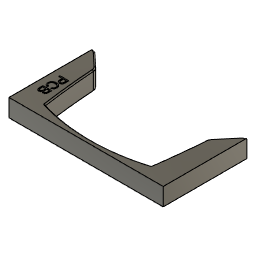
pcb_Dispensor_holder (Autodesk Fusion 360 design; units mm, degrees)
Autodesk Fusion 360 part; units mm, degrees
sketch "Sketch1" plane through (0, 0, 0) normal (0, 0, 1) x (1, 0, 0)
  line L0 (0, 0) -> (70, 0)
  line L1 (70, 0) -> (70, 70)
  line L2 (70, 70) -> (0, 70)
  line L3 (0, 70) -> (0, 0)
  line L4 (35, 0) -> (35, 2)
  spline S0 degree 5 poles (10.999997, 5.500001) (11.155561, 5.453683) (11.466888, 5.361799) (11.934471, 5.226228) (12.559102, 5.049976) (13.341865, 4.83719) (14.126594, 4.631952) (14.913263, 4.43428) (15.70183, 4.244194) (16.492223, 4.061708) (17.284358, 3.886836) (18.078142, 3.719588) (18.873486, 3.559975) (19.670315, 3.408007) (20.468575, 3.263698) (21.268224, 3.127064) (22.069221, 2.998132) (22.871516, 2.876939) (23.675037, 2.76354) (24.479682, 2.658009) (25.285329, 2.560422) (26.091853, 2.470835) (26.899136, 2.389272) (27.707084, 2.3157) (28.515633, 2.250011) (29.324747, 2.192062) (30.134393, 2.141705) (30.944536, 2.098828) (31.755125, 2.063387) (32.566073, 2.035442) (33.377278, 2.015122) (34.188626, 2.002585) (35.000008, 1.997988) (35.811324, 2.001442) (36.622501, 2.012982) (37.433482, 2.032584) (38.244219, 2.060187) (39.054663, 2.095711) (39.864763, 2.139079) (40.674451, 2.190236) (41.483649, 2.249147) (42.292272, 2.315789) (43.100227, 2.390151) (43.907418, 2.472228) (44.713752, 2.562017) (45.519136, 2.659519) (46.323491, 2.764743) (47.126755, 2.877707) (47.928887, 2.998437) (48.729875, 3.126975) (49.529715, 3.263365) (50.328395, 3.407636) (51.125872, 3.559798) (51.922055, 3.719827) (52.716787, 3.887649) (53.509869, 4.063161) (54.301082, 4.246242) (55.090222, 4.436771) (55.877114, 4.634637) (56.661648, 4.839761) (57.443758, 5.052087) (58.067484, 5.227679) (58.534171, 5.36259) (58.844804, 5.453959) (58.999997, 5.500001) knots 0 0 0 0 0 0 0.01666667 0.03333333 0.05 0.06666667 0.08333333 0.1 0.11666667 0.13333333 0.15 0.16666667 0.18333333 0.2 0.21666667 0.23333333 0.25 0.26666667 0.28333333 0.3 0.31666667 0.33333333 0.35 0.36666667 0.38333333 0.4 0.41666667 0.43333333 0.45 0.46666667 0.48333333 0.5 0.51666667 0.53333333 0.55 0.56666667 0.58333333 0.6 0.61666667 0.63333333 0.65 0.66666667 0.68333333 0.7 0.71666667 0.73333333 0.75 0.76666667 0.78333333 0.8 0.81666667 0.83333333 0.85 0.86666667 0.88333333 0.9 0.91666667 0.93333333 0.95 0.96666667 0.98333333 1 1 1 1 1 1
  spline S1 degree 5 poles (58.999997, 5.500001) (59.01455, 5.602527) (59.04395, 5.810642) (59.088931, 6.131994) (59.150678, 6.578903) (59.230393, 7.164734) (59.311475, 7.767981) (59.391329, 8.366775) (59.466575, 8.932747) (59.535207, 9.449558) (59.598272, 9.92737) (59.66196, 10.420796) (59.73467, 11.003713) (59.824179, 11.745021) (59.934208, 12.679149) (60.063255, 13.795991) (60.206503, 15.057047) (60.356952, 16.404923) (60.506823, 17.775214) (60.64889, 19.107692) (60.777733, 20.356871) (60.891317, 21.505277) (60.990565, 22.559989) (61.078304, 23.543942) (61.158448, 24.48917) (61.235067, 25.429138) (61.311554, 26.391886) (61.389627, 27.391781) (61.469549, 28.431304) (61.550566, 29.504582) (61.631253, 30.600245) (61.709907, 31.704562) (61.784901, 32.804352) (61.855087, 33.890205) (61.919728, 34.956001) (61.978402, 35.998148) (62.020415, 36.811581) (62.049133, 37.41002) (62.067038, 37.803816) (62.075682, 37.999422) knots 0 0 0 0 0 0 0.02857143 0.05714286 0.08571429 0.11428571 0.14285714 0.17142857 0.2 0.22857143 0.25714286 0.28571429 0.31428571 0.34285714 0.37142857 0.4 0.42857143 0.45714286 0.48571429 0.51428571 0.54285714 0.57142857 0.6 0.62857143 0.65714286 0.68571429 0.71428571 0.74285714 0.77142857 0.8 0.82857143 0.85714286 0.88571429 0.91428571 0.94285714 0.97142857 1 1 1 1 1 1
  spline S2 degree 5 poles (10.999997, 5.500001) (10.95489, 5.823121) (10.865295, 6.469506) (10.732765, 7.439517) (10.559793, 8.733734) (10.349927, 10.352962) (10.146623, 11.973629) (9.950184, 13.595674) (9.761002, 15.218964) (9.579547, 16.843273) (9.406299, 18.468328) (9.241664, 20.093857) (9.085891, 21.719638) (8.938976, 23.345548) (8.800554, 24.971608) (8.670024, 26.597942) (8.546659, 28.224733) (8.429709, 29.85218) (8.318502, 31.480453) (8.212533, 33.109654) (8.111452, 34.739832) (8.034323, 36.044766) (7.978526, 37.023912) (7.942236, 37.676872) (7.924318, 38.003401) knots 0 0 0 0 0 0 0.05 0.1 0.15 0.2 0.25 0.3 0.35 0.4 0.45 0.5 0.55 0.6 0.65 0.7 0.75 0.8 0.85 0.9 0.95 1 1 1 1 1 1
  line L5 (7.924318, 38.003401) -> (0, 38.003401)
  line L6 (62.075682, 37.999422) -> (70, 37.999422)
  point P0 (18.873057, 3.562043)
  point P1 (14.913459, 4.436245)
  point P2 (30.944166, 2.100711)
  point P3 (22.870856, 2.879029)
  point P4 (43.099861, 2.392063)
  point P5 (51.125881, 3.56183)
  point P6 (26.89909, 2.39129)
  point P7 (39.054312, 2.097659)
  point P8 (35, 2)
  point P9 (55.093436, 4.439536)
  point P10 (47.126108, 2.879595)
  point P11 (61.715357, 31.79493)
  point P12 (9.087814, 21.72277)
  point P13 (9.952125, 13.594921)
  point P14 (8.43127, 29.85062)
  point P15 (59.536775, 9.462231)
  point P16 (60.67846, 19.401486)
  point P17 (59.272705, 7.480264)
  point P18 (59.787881, 11.447136)
  point P19 (61.247514, 25.590178)
  dimension "d2" = 70
  dimension "d3" = 70
  dimension "d4" = 2
  constraint horizontal L0
  constraint vertical L1
  constraint horizontal L2
  constraint vertical L3
  constraint coincident L0.start L3.end
  constraint midpoint L0 L4.start
  constraint perpendicular L0 L4
  constraint perpendicular L3 L5
  constraint perpendicular L1 L6
  constraint equal L5 L6
  measures "d2" distance of L0.start L0.end
  measures "d3" distance of L0.start L2.end
  measures "d4" distance of L4.start P8
extrude "Extrude1" add sketch "Sketch1" along normal blind 8 contours L0 L3 L4 S0 S2 L5 | L0 L1 L4 S0 S1 L6 picked at (3.666666, 14.501134) picked at (66.333332, 14.499808)
chamfer "Chamfer1" distance 7 distance2 9 1 edges at (62.075682, 37.999422, 4) measured on face at (64.717121, 37.999422, 2.666667)
chamfer "Chamfer1" distance 7 distance2 7 1 edges at (7.924318, 38.003401, 4) measured on face at (9.188265, 20.663801, 6)
fillet "Fillet1" radius 3 4 edges at (69.075682, 37.999422, 4) (61.513537, 29.016995, 4) (8.350994, 31.016417, 4) (0.924318, 38.003401, 4)
fillet "Fillet2" radius 0.5 9 edges at (34.999992, 2, 8) (0.95535, 37.750746, 8) (4.635654, 34.511792, 8) (8.149345, 30.922984, 8) (9.49426, 17.653194, 8) (60.042115, 13.616714, 8) (61.654743, 28.96036, 8) (65.174872, 33.365983, 8) (69.015881, 37.645309, 8)
sketch "Sketch2" plane through (0, 0, 8) normal (0, 0, 1) x (-1, 0, 0)
  line L0 (0, -37.500788) -> (0, 0)
  line L1 (0, 0) -> (-70, 0)
  line L2 (-70, 0) -> (-70, -37.490585)
  spline S0 degree 3 poles (-68.59563, -36.652856) (-68.783694, -36.87624) (-69.011266, -37.066303) (-69.492981, -37.342508) (-69.742224, -37.437076) (-70, -37.490585) knots 0 0 0 0 0.08760236 0.08760236 0.16658474 0.16658474 0.16658474 0.16658474
  line L3 (-62.519109, -29.435075) -> (-68.59563, -36.652856)
  spline S1 degree 3 poles (-61.938909, -28.016044) (-61.959496, -28.284633) (-62.023868, -28.549832) (-62.226006, -29.028259) (-62.3581, -29.243826) (-62.519109, -29.435075) knots 0 0 0 0 0.080813 0.080813 0.155813 0.155813 0.155813 0.155813
  spline S2 degree 3 poles (-59.449928, -5.111943) (-59.464964, -5.217874) (-59.479999, -5.323804) (-59.495035, -5.429734) (-59.73744, -7.137512) (-59.968364, -8.847014) (-60.356187, -11.944064) (-60.514111, -13.331475) (-60.827694, -16.106506) (-60.980694, -17.494467) (-61.447016, -21.922745) (-61.705327, -24.968565) (-61.938909, -28.016044) knots -2.30429934 -2.30429934 -2.30429934 -2.30429934 -2.27220171 -2.27220171 -2.27220171 -1.75473297 -1.75473297 -1.33582908 -1.33582908 -0.91692518 -0.91692518 0 0 0 0
  spline S3 degree 3 poles (-10.54924, -5.112517) (-10.651933, -5.081941) (-10.754625, -5.051366) (-10.857317, -5.02079) (-14.768037, -3.856418) (-18.762955, -2.973769) (-26.838164, -1.794213) (-30.919265, -1.502845) (-34.999643, -1.5) (-39.080099, -1.497155) (-43.160271, -1.797009) (-51.236861, -2.972737) (-55.230276, -3.860084) (-59.142208, -5.020651) (-59.244781, -5.051082) (-59.347354, -5.081513) (-59.449928, -5.111943) knots -4.92864568 -4.92864568 -4.92864568 -4.92864568 -4.89650146 -4.89650146 -4.89650146 -3.67238774 -3.67238774 -2.44827402 -2.44827402 -2.44827402 -1.22413701 -1.22413701 0 0 0 0.03209763 0.03209763 0.03209763 0.03209763
  spline S4 degree 3 poles (-7.932748, -29.812036) (-8.218624, -25.735112) (-8.56417, -21.662087) (-9.430424, -13.534173) (-9.939748, -9.478557) (-10.504799, -5.430872) (-10.519612, -5.324753) (-10.534426, -5.218635) (-10.54924, -5.112517) knots -2.45216078 -2.45216078 -2.45216078 -2.45216078 -1.22608039 -1.22608039 0 0 0 0.03214422 0.03214422 0.03214422 0.03214422
  spline S5 degree 3 poles (-7.151916, -31.45801) (-7.265096, -31.35153) (-7.368324, -31.234463) (-7.60618, -30.907834) (-7.722314, -30.684882) (-7.873835, -30.244018) (-7.917533, -30.029023) (-7.932748, -29.812036) knots 0 0 0 0 0.04661863 0.04661863 0.12120843 0.12120843 0.18646451 0.18646451 0.18646451 0.18646451
  line L4 (-1.434175, -36.837236) -> (-7.151916, -31.45801)
  spline S6 degree 3 poles (0, -37.500788) (-0.284132, -37.468895) (-0.562702, -37.387784) (-1.044127, -37.152317) (-1.25209, -37.008541) (-1.434175, -36.837236) knots 0.00467237 0.00467237 0.00467237 0.00467237 0.09044877 0.09044877 0.16544877 0.16544877 0.16544877 0.16544877
  line L5 (-3.028265, -20.094822) -> (-7.028264, -20.098258)
  line L6 (-7.028264, -20.098258) -> (-7.02956, -18.589391)
  spline S7 degree 2 poles (-7.02956, -18.589391) (-7.029902, -18.191028) (-6.991883, -17.9809) knots 0 0 0 1 1 1
  spline S8 degree 2 poles (-6.991883, -17.9809) (-6.943023, -17.686179) (-6.805405, -17.486879) knots 0 0 0 1 1 1
  spline S9 degree 2 poles (-6.805405, -17.486879) (-6.667786, -17.287579) (-6.419596, -17.165947) knots 0 0 0 1 1 1
  spline S10 degree 2 poles (-6.419596, -17.165947) (-6.171405, -17.044315) (-5.873998, -17.044059) knots 0 0 0 1 1 1
  spline S11 degree 2 poles (-5.873998, -17.044059) (-5.363766, -17.043621) (-5.010145, -17.368011) knots 0 0 0 1 1 1
  spline S12 degree 2 poles (-5.010145, -17.368011) (-4.656523, -17.6924) (-4.655794, -18.540967) knots 0 0 0 1 1 1
  line L7 (-4.655794, -18.540967) -> (-4.654913, -19.566888)
  line L8 (-4.654913, -19.566888) -> (-3.02872, -19.565491)
  line L9 (-3.02872, -19.565491) -> (-3.028265, -20.094822)
  line L10 (-5.126946, -19.567293) -> (-5.127834, -18.533187)
  spline S13 degree 2 poles (-5.127834, -18.533187) (-5.128275, -18.020227) (-5.319456, -17.804838) knots 0 0 0 1 1 1
  spline S14 degree 2 poles (-5.319456, -17.804838) (-5.510637, -17.58945) (-5.857157, -17.589748) knots 0 0 0 1 1 1
  spline S15 degree 2 poles (-5.857157, -17.589748) (-6.108181, -17.589963) (-6.286789, -17.716993) knots 0 0 0 1 1 1
  spline S16 degree 2 poles (-6.286789, -17.716993) (-6.465398, -17.844022) (-6.522518, -18.051438) knots 0 0 0 1 1 1
  spline S17 degree 2 poles (-6.522518, -18.051438) (-6.557874, -18.185166) (-6.557565, -18.545329) knots 0 0 0 1 1 1
  line L11 (-6.557565, -18.545329) -> (-6.556686, -19.568521)
  line L12 (-6.556686, -19.568521) -> (-5.126946, -19.567293)
  line L13 (-4.436374, -13.514856) -> (-4.303132, -12.98541)
  spline S18 degree 2 poles (-4.303132, -12.98541) (-3.650874, -13.151289) (-3.308075, -13.583464) knots 0 0 0 1 1 1
  spline S19 degree 2 poles (-3.308075, -13.583464) (-2.965275, -14.015639) (-2.964738, -14.640468) knots 0 0 0 1 1 1
  spline S20 degree 2 poles (-2.964738, -14.640468) (-2.964182, -15.287125) (-3.227136, -15.692535) knots 0 0 0 1 1 1
  spline S21 degree 2 poles (-3.227136, -15.692535) (-3.490089, -16.097946) (-3.989225, -16.309834) knots 0 0 0 1 1 1
  spline S22 degree 2 poles (-3.989225, -16.309834) (-4.488361, -16.521723) (-5.061349, -16.522215) knots 0 0 0 1 1 1
  spline S23 degree 2 poles (-5.061349, -16.522215) (-5.686178, -16.522752) (-6.151594, -16.284407) knots 0 0 0 1 1 1
  spline S24 degree 2 poles (-6.151594, -16.284407) (-6.617011, -16.046061) (-6.858863, -15.605614) knots 0 0 0 1 1 1
  spline S25 degree 2 poles (-6.858863, -15.605614) (-7.100714, -15.165167) (-7.101169, -14.635836) knots 0 0 0 1 1 1
  spline S26 degree 2 poles (-7.101169, -14.635836) (-7.101685, -14.035563) (-6.796443, -13.626023) knots 0 0 0 1 1 1
  spline S27 degree 2 poles (-6.796443, -13.626023) (-6.491201, -13.216485) (-5.937452, -13.055026) knots 0 0 0 1 1 1
  line L14 (-5.937452, -13.055026) -> (-5.814221, -13.576067)
  spline S28 degree 2 poles (-5.814221, -13.576067) (-6.250663, -13.715596) (-6.449617, -13.980433) knots 0 0 0 1 1 1
  spline S29 degree 2 poles (-6.449617, -13.980433) (-6.648571, -14.245269) (-6.648227, -14.646361) knots 0 0 0 1 1 1
  spline S30 degree 2 poles (-6.648227, -14.646361) (-6.647831, -15.107479) (-6.426555, -15.416976) knots 0 0 0 1 1 1
  spline S31 degree 2 poles (-6.426555, -15.416976) (-6.20528, -15.726472) (-5.83273, -15.851663) knots 0 0 0 1 1 1
  spline S32 degree 2 poles (-5.83273, -15.851663) (-5.46018, -15.976855) (-5.064546, -15.976515) knots 0 0 0 1 1 1
  spline S33 degree 2 poles (-5.064546, -15.976515) (-4.554314, -15.976077) (-4.173814, -15.827046) knots 0 0 0 1 1 1
  spline S34 degree 2 poles (-4.173814, -15.827046) (-3.793315, -15.678015) (-3.605317, -15.364075) knots 0 0 0 1 1 1
  spline S35 degree 2 poles (-3.605317, -15.364075) (-3.417319, -15.050134) (-3.417633, -14.684513) knots 0 0 0 1 1 1
  spline S36 degree 2 poles (-3.417633, -14.684513) (-3.418015, -14.239766) (-3.67476, -13.931664) knots 0 0 0 1 1 1
  spline S37 degree 2 poles (-3.67476, -13.931664) (-3.931506, -13.623562) (-4.436374, -13.514856) knots 0 0 0 1 1 1
  line L15 (-3.034915, -12.354034) -> (-7.034914, -12.35747)
  line L16 (-7.034914, -12.35747) -> (-7.036203, -10.856788)
  spline S38 degree 2 poles (-7.036203, -10.856788) (-7.036596, -10.398399) (-6.915416, -10.12135) knots 0 0 0 1 1 1
  spline S39 degree 2 poles (-6.915416, -10.12135) (-6.794235, -9.844301) (-6.541982, -9.687195) knots 0 0 0 1 1 1
  spline S40 degree 2 poles (-6.541982, -9.687195) (-6.289729, -9.53009) (-6.01415, -9.529853) knots 0 0 0 1 1 1
  spline S41 degree 2 poles (-6.01415, -9.529853) (-5.75767, -9.529632) (-5.531084, -9.668591) knots 0 0 0 1 1 1
  spline S42 degree 2 poles (-5.531084, -9.668591) (-5.304497, -9.807552) (-5.165102, -10.088468) knots 0 0 0 1 1 1
  spline S43 degree 2 poles (-5.165102, -10.088468) (-5.059002, -9.725485) (-4.802689, -9.530176) knots 0 0 0 1 1 1
  spline S44 degree 2 poles (-4.802689, -9.530176) (-4.546377, -9.334867) (-4.197127, -9.334567) knots 0 0 0 1 1 1
  spline S45 degree 2 poles (-4.197127, -9.334567) (-3.91609, -9.334326) (-3.674515, -9.452808) knots 0 0 0 1 1 1
  spline S46 degree 2 poles (-3.674515, -9.452808) (-3.43294, -9.571291) (-3.301821, -9.745803) knots 0 0 0 1 1 1
  spline S47 degree 2 poles (-3.301821, -9.745803) (-3.170703, -9.920316) (-3.103628, -10.183559) knots 0 0 0 1 1 1
  spline S48 degree 2 poles (-3.103628, -10.183559) (-3.036553, -10.446804) (-3.036225, -10.828795) knots 0 0 0 1 1 1
  line L17 (-3.036225, -10.828795) -> (-3.034915, -12.354034)
  line L18 (-5.354605, -11.826694) -> (-5.355348, -10.961756)
  spline S49 degree 2 poles (-5.355348, -10.961756) (-5.35565, -10.609778) (-5.402166, -10.457021) knots 0 0 0 1 1 1
  spline S50 degree 2 poles (-5.402166, -10.457021) (-5.462367, -10.255163) (-5.601609, -10.152963) knots 0 0 0 1 1 1
  spline S51 degree 2 poles (-5.601609, -10.152963) (-5.740851, -10.050764) (-5.950946, -10.050945) knots 0 0 0 1 1 1
  spline S52 degree 2 poles (-5.950946, -10.050945) (-6.150128, -10.051116) (-6.301478, -10.146743) knots 0 0 0 1 1 1
  spline S53 degree 2 poles (-6.301478, -10.146743) (-6.452828, -10.242372) (-6.50861, -10.419772) knots 0 0 0 1 1 1
  spline S54 degree 2 poles (-6.50861, -10.419772) (-6.564393, -10.597174) (-6.564022, -11.028279) knots 0 0 0 1 1 1
  line L19 (-6.564022, -11.028279) -> (-6.563336, -11.827733)
  line L20 (-6.563336, -11.827733) -> (-5.354605, -11.826694)
  line L21 (-3.507402, -11.825108) -> (-3.508258, -10.829201)
  spline S55 degree 2 poles (-3.508258, -10.829201) (-3.508478, -10.572721) (-3.527667, -10.469053) knots 0 0 0 1 1 1
  spline S56 degree 2 poles (-3.527667, -10.469053) (-3.560566, -10.286272) (-3.63707, -10.163554) knots 0 0 0 1 1 1
  spline S57 degree 2 poles (-3.63707, -10.163554) (-3.713574, -10.040837) (-3.859617, -9.961836) knots 0 0 0 1 1 1
  spline S58 degree 2 poles (-3.859617, -9.961836) (-4.00566, -9.882834) (-4.196656, -9.882998) knots 0 0 0 1 1 1
  spline S59 degree 2 poles (-4.196656, -9.882998) (-4.420394, -9.88319) (-4.58537, -9.997929) knots 0 0 0 1 1 1
  spline S60 degree 2 poles (-4.58537, -9.997929) (-4.750347, -10.112669) (-4.817021, -10.316001) knots 0 0 0 1 1 1
  spline S61 degree 2 poles (-4.817021, -10.316001) (-4.883695, -10.519332) (-4.883367, -10.901324) knots 0 0 0 1 1 1
  line L22 (-4.883367, -10.901324) -> (-4.882572, -11.826289)
  line L23 (-4.882572, -11.826289) -> (-3.507402, -11.825108)
extrude "Extrude2" cut sketch "Sketch2" against normal blind 1 contours L5 L6 S7 S8 S9 S10 S11 S12 L7 L8 L9 | L13 S18 S19 S20 S21 S22 S23 S24 S25 S26 S27 L14 S28 S29 S30 S31 S32 S33 S34 S35 S36 S37 | L15 L16 S38 S39 S40 S41 S42 S43 S44 S45 S46 S47 S48 L17 picked at (-5.061158, -19.920124) picked at (-5.282425, -16.327013) picked at (-4.984134, -12.179264)
equation "box_width = 70 mm"
equation "d2 = box_width"
equation "d3 = box_width"
